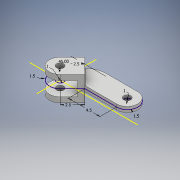
# Autodesk Inventor part: 7c
Saved by Autodesk Inventor 2018 (Build 220112000, 112)
## iProperties
Created: 2018-10-23
Part Number: 7c
Material: Generic
Document SubType Name: Modeling
Designer: Jerry
Density: 1 g/cm^3
Appearance: Default
Author: Jerry
Autodesk Inventor part; units mm, degrees
ref_plane "YZ Plane" through (0, 0, 0) normal (1, 0, 0) x (0, 1, 0)
ref_plane "XZ Plane" through (0, 0, 0) normal (0, 1, 0) x (-1, 0, 0)
ref_plane "XY Plane" through (0, 0, 0) normal (0, 0, 1) x (1, 0, 0)
sketch "Sketch1" plane through (0, 0, 0) normal (0, 0, 1) x (1, 0, 0)
  line L0 (0, -3.3292) -> (0, 5.126) projected
  line L1 (-4.3113, 0) -> (11.0184, 0) projected
  line L2 (-1.0607, 1.0607) -> (0.7071, 2.8284)
  arc A0 (2.8284, 3.7071) -> (0.7071, 2.8284) centre (2.8284, 0.7071) ccw
  line L3 (2.8284, 3.7071) -> (7.3284, 3.7071)
  arc A1 (7.3284, 0.7071) -> (7.3284, 3.7071) centre (7.3284, 2.2071) ccw
  line L4 (7.3284, 0.7071) -> (2.8284, 0.7071)
  line L5 (2.8284, 0.7071) -> (1.0607, -1.0607)
  arc A2 (-1.0607, 1.0607) -> (1.0607, -1.0607) centre (0, 0) ccw
  circle A3 centre (0, 0) radius 0.5
  circle A4 centre (7.3284, 2.2071) radius 0.5
  line L6 (2.8284, 0.7071) -> (0.7071, 2.8284)
  line L7 (2.2981, 0.1768) -> (0.1768, 2.2981)
  line L8 (2.2981, 0.1768) -> (2.2981, 0.1768)
  dimension "d0" = 4.5
  dimension "d1" = 45
  dimension "d2" = 1
  dimension "d3" = 1
  dimension "d5" = 2.5
  dimension "d6" = 1.5
  dimension "d8" = 2.5
  dimension "d9" = 1.5
  constraints: 14 end point, 6 point on circle, 6 tangent, 5 centre point, 5 coincident, 3 point on line, 2 parallel, 1 horizontal, 1 perpendicular, 1 other
  measures "d0" distance of L4.start L4.end
  measures "d1" angle of L2 L3
  measures "d2" diameter of A4
  measures "d3" diameter of A3
  measures "d5" distance of L5.end L4.end
  measures "d6" radius of A1
  measures "d8" distance of L2.start L2.end
  measures "d9" radius of A2
extrude "Extrusion1" add sketch "Sketch1" along normal mid plane 0.75 contours L6 A0 L3 A1 L4
extrude "Extrusion2" add sketch "Sketch1" along normal mid plane 3.5 contours L7 L2 L6 L5
extrude "Extrusion3" add sketch "Sketch1" along normal mid plane 3.5 contours A2 L1 A3 L0 | L0 A3 L1 L5 A2 | A2 L2 L0 A3 L1 | A3 L0 L2 L7 L5 L1
extrude "Extrusion4" cut sketch "Sketch1" along normal mid plane 2 contours A2 L1 A3 L0 | L0 A3 L1 L5 A2 | A2 L2 L0 A3 L1 | A3 L0 L2 L7 L5 L1
fillet "Fillet1" radius 0.1 2 edges at (1.7678, 1.7678, 0.375) (1.7678, 1.7678, -0.375)
body "Solid1"
